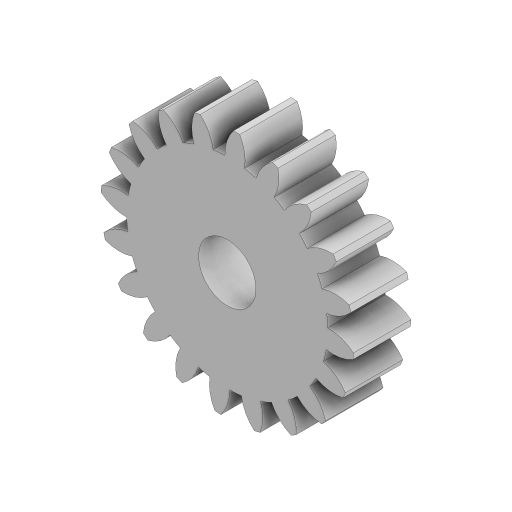
# Autodesk Inventor part: ENGRANAJE PARA RODILLO
Saved by Autodesk Inventor 2024 (Build 280153000, 153)
## iProperties
Created: 2024-06-28
Part Number: ENGRANAJE PARA RODILLO
Material: Generic
Document SubType Name: Modeling
Designer: Jhuliams
Density: 1 g/cm^3
Appearance: Default
Author: Jhuliams
Autodesk Inventor part; units mm, degrees
ref_plane "YZ Plane" through (0, 0, 0) normal (1, 0, 0) x (0, 1, 0)
ref_plane "XZ Plane" through (0, 0, 0) normal (0, 1, 0) x (-1, 0, 0)
ref_plane "XY Plane" through (0, 0, 0) normal (0, 0, 1) x (1, 0, 0)
sketch "Sketch1" plane through (0, 0, 0) normal (0, 0, 1) x (1, 0, 0)
  arc A0 (21.8933, -2.1639) -> (21.9716, -1.1171) centre (0, 0) ccw
  circle A1 centre (0, 0) radius 17.5
  line L0 (0, 0) -> (28.7195, 0) construction
  arc A2 (21.9716, -1.1171) -> (17.4952, 0.4105) centre (17.6604, -6.4279) ccw
  line L1 (0, 0) -> (30.5019, 0) construction
  arc A3 (17.2394, -3.0086) -> (21.8933, -2.1639) centre (18.4202, 3.7291) ccw
  arc A4 (21.4905, 4.7074) -> (21.2414, 5.7272) centre (0, 0) ccw
  arc A5 (21.2414, 5.7272) -> (16.512, 5.7967) centre (18.7824, -0.6559) ccw
  arc A6 (17.3254, 2.4659) -> (21.4905, 4.7074) centre (16.3662, 9.2388) ccw
  arc A7 (18.984, 11.1179) -> (18.432, 12.0109) centre (0, 0) ccw
  arc A8 (18.432, 12.0109) -> (13.9126, 10.6155) centre (18.0658, 5.1803) ccw
  arc A9 (15.7154, 7.6991) -> (18.984, 11.1179) centre (12.7103, 13.844) ccw
  arc A10 (14.6192, 16.4401) -> (13.8183, 17.1188) centre (0, 0) ccw
  arc A11 (13.8183, 17.1188) -> (9.9513, 14.3952) centre (15.5808, 10.5094) ccw
  arc A12 (12.5671, 12.1786) -> (14.6192, 16.4401) centre (7.8102, 17.0942) ccw
  arc A13 (8.8234, 20.1531) -> (7.852, 20.5511) centre (0, 0) ccw
  arc A14 (7.852, 20.5511) -> (5.0159, 16.7658) centre (11.5707, 14.8098) ccw
  arc A15 (8.1886, 15.466) -> (8.8234, 20.1531) centre (2.1455, 18.671) ccw
  arc A16 (2.1639, 21.8933) -> (1.1171, 21.9716) centre (0, 0) ccw
  arc A17 (1.1171, 21.9716) -> (-0.4105, 17.4952) centre (6.4279, 17.6604) ccw
  arc A18 (3.0086, 17.2394) -> (2.1639, 21.8933) centre (-3.7291, 18.4202) ccw
  arc A19 (-4.7074, 21.4905) -> (-5.7272, 21.2414) centre (0, 0) ccw
  arc A20 (-5.7272, 21.2414) -> (-5.7967, 16.512) centre (0.6559, 18.7824) ccw
  arc A21 (-2.4659, 17.3254) -> (-4.7074, 21.4905) centre (-9.2388, 16.3662) ccw
  arc A22 (-11.1179, 18.984) -> (-12.0109, 18.432) centre (0, 0) ccw
  arc A23 (-12.0109, 18.432) -> (-10.6155, 13.9126) centre (-5.1803, 18.0658) ccw
  arc A24 (-7.6991, 15.7154) -> (-11.1179, 18.984) centre (-13.844, 12.7103) ccw
  arc A25 (-16.4401, 14.6192) -> (-17.1188, 13.8183) centre (0, 0) ccw
  arc A26 (-17.1188, 13.8183) -> (-14.3952, 9.9513) centre (-10.5094, 15.5808) ccw
  arc A27 (-12.1786, 12.5671) -> (-16.4401, 14.6192) centre (-17.0942, 7.8102) ccw
  arc A28 (-20.1531, 8.8234) -> (-20.5511, 7.852) centre (0, 0) ccw
  arc A29 (-20.5511, 7.852) -> (-16.7658, 5.0159) centre (-14.8098, 11.5707) ccw
  arc A30 (-15.466, 8.1886) -> (-20.1531, 8.8234) centre (-18.671, 2.1455) ccw
  arc A31 (-21.8933, 2.1639) -> (-21.9716, 1.1171) centre (0, 0) ccw
  arc A32 (-21.9716, 1.1171) -> (-17.4952, -0.4105) centre (-17.6604, 6.4279) ccw
  arc A33 (-17.2394, 3.0086) -> (-21.8933, 2.1639) centre (-18.4202, -3.7291) ccw
  arc A34 (-21.4905, -4.7074) -> (-21.2414, -5.7272) centre (0, 0) ccw
  arc A35 (-21.2414, -5.7272) -> (-16.512, -5.7967) centre (-18.7824, 0.6559) ccw
  arc A36 (-17.3254, -2.4659) -> (-21.4905, -4.7074) centre (-16.3662, -9.2388) ccw
  arc A37 (-18.984, -11.1179) -> (-18.432, -12.0109) centre (0, 0) ccw
  arc A38 (-18.432, -12.0109) -> (-13.9126, -10.6155) centre (-18.0658, -5.1803) ccw
  arc A39 (-15.7154, -7.6991) -> (-18.984, -11.1179) centre (-12.7103, -13.844) ccw
  arc A40 (-14.6192, -16.4401) -> (-13.8183, -17.1188) centre (0, 0) ccw
  arc A41 (-13.8183, -17.1188) -> (-9.9513, -14.3952) centre (-15.5808, -10.5094) ccw
  arc A42 (-12.5671, -12.1786) -> (-14.6192, -16.4401) centre (-7.8102, -17.0942) ccw
  arc A43 (-8.8234, -20.1531) -> (-7.852, -20.5511) centre (0, 0) ccw
  arc A44 (-7.852, -20.5511) -> (-5.0159, -16.7658) centre (-11.5707, -14.8098) ccw
  arc A45 (-8.1886, -15.466) -> (-8.8234, -20.1531) centre (-2.1455, -18.671) ccw
  arc A46 (-2.1639, -21.8933) -> (-1.1171, -21.9716) centre (0, 0) ccw
  arc A47 (-1.1171, -21.9716) -> (0.4105, -17.4952) centre (-6.4279, -17.6604) ccw
  arc A48 (-3.0086, -17.2394) -> (-2.1639, -21.8933) centre (3.7291, -18.4202) ccw
  arc A49 (4.7074, -21.4905) -> (5.7272, -21.2414) centre (0, 0) ccw
  arc A50 (5.7272, -21.2414) -> (5.7967, -16.512) centre (-0.6559, -18.7824) ccw
  arc A51 (2.4659, -17.3254) -> (4.7074, -21.4905) centre (9.2388, -16.3662) ccw
  arc A52 (11.1179, -18.984) -> (12.0109, -18.432) centre (0, 0) ccw
  arc A53 (12.0109, -18.432) -> (10.6155, -13.9126) centre (5.1803, -18.0658) ccw
  arc A54 (7.6991, -15.7154) -> (11.1179, -18.984) centre (13.844, -12.7103) ccw
  arc A55 (16.4401, -14.6192) -> (17.1188, -13.8183) centre (0, 0) ccw
  arc A56 (17.1188, -13.8183) -> (14.3952, -9.9513) centre (10.5094, -15.5808) ccw
  arc A57 (12.1786, -12.5671) -> (16.4401, -14.6192) centre (17.0942, -7.8102) ccw
  arc A58 (20.1531, -8.8234) -> (20.5511, -7.852) centre (0, 0) ccw
  arc A59 (20.5511, -7.852) -> (16.7658, -5.0159) centre (14.8098, -11.5707) ccw
  arc A60 (15.466, -8.1886) -> (20.1531, -8.8234) centre (18.671, -2.1455) ccw
  point P0 (16.7658, -5.0159)
  point P1 (17.2394, -3.0086)
  point P2 (17.3254, 2.4659)
  point P3 (16.512, 5.7967)
  point P4 (13.9126, 10.6155)
  point P5 (12.5671, 12.1786)
  point P6 (9.9513, 14.3952)
  point P7 (5.0159, 16.7658)
  point P8 (3.0086, 17.2394)
  point P9 (-0.4105, 17.4952)
  point P10 (-2.4659, 17.3254)
  point P11 (-5.7967, 16.512)
  point P12 (-10.6155, 13.9126)
  point P13 (-12.1786, 12.5671)
  point P14 (-14.3952, 9.9513)
  point P15 (-16.7658, 5.0159)
  point P16 (-17.2394, 3.0086)
  point P17 (-17.4952, -0.4105)
  point P18 (-17.3254, -2.4659)
  point P19 (-16.512, -5.7967)
  point P20 (-13.9126, -10.6155)
  point P21 (-12.5671, -12.1786)
  point P22 (-9.9513, -14.3952)
  point P23 (-8.1886, -15.466)
  point P24 (-3.0086, -17.2394)
  point P25 (0.4105, -17.4952)
  point P26 (2.4659, -17.3254)
  point P27 (5.7967, -16.512)
  point P28 (10.6155, -13.9126)
  point P29 (12.1786, -12.5671)
  point P30 (15.466, -8.1886)
  dimension "d13" = 35
  dimension "d12" = 44
  dimension "d18" = 360
  constraints: 120 point on circle, 60 centre point, 4 end point, 2 horizontal, 1 coincident, 204 other
  measures "d12" diameter of A0
extrude "Extrusion1" add sketch "Sketch1" along normal blind 10
sketch "Sketch2" plane through (0, 0, 10) normal (0, 0, 1) x (1, 0, 0)
  circle A0 centre (0, 0) radius 5
  dimension "d20" = 10
  constraints: 1 centre point, 1 coincident
  measures "d20" diameter of A0
extrude "Extrusion2" cut sketch "Sketch2" against normal blind 10
body "Solid1"
